mpu6050 (Autodesk Fusion 360 design; units mm, degrees)
Autodesk Fusion 360 part; units mm, degrees
sketch "Sketch1" plane through (0, 0, 0) normal (0, 0, 1) x (1, 0, 0)
  line L0 (-8.25, -9.75) -> (8.25, -9.75)
  line L1 (8.25, -9.75) -> (8.25, 9.75)
  line L2 (8.25, 9.75) -> (-8.25, 9.75)
  line L3 (-8.25, 9.75) -> (-8.25, -9.75)
  line L4 (-8.25, -9.75) -> (8.25, 9.75) construction
  line L5 (8.25, -9.75) -> (-8.25, 9.75) construction
  line L6 (-6.25, 9.75) -> (-6.25, -9.75) construction
  line L7 (-3.25, 9.75) -> (-3.25, -9.75) construction
  line L8 (-3.25, 0) -> (-6.25, 0) construction
  line L9 (-4.75, 7.25) -> (-4.75, -7.25) construction
  circle A0 centre (-4.75, 7.25) radius 1.5
  line L10 (-4.75, 7.25) -> (-4.75, 9.75) construction
  circle A1 centre (-4.75, -7.25) radius 1.5
  dimension "d1" = 16.5
  dimension "d2" = 19.5
  dimension "d3" = 2
  dimension "d4" = 3
  dimension "d5" = 2.5
  constraint horizontal L0
  constraint perpendicular L0 L1
  constraint parallel L0 L2
  constraint parallel L1 L3
  constraint coincident L4 origin
  constraint coincident L5 origin
  constraint coincident L2 L6.start
  constraint coincident L0 L6.end
  constraint perpendicular L0 L6
  constraint coincident L2 L7.start
  constraint coincident L0 L7.end
  constraint perpendicular L0 L7
  constraint midpoint L7 L8.start
  constraint midpoint L6 L8.end
  constraint perpendicular L8 L9
  constraint midpoint L8 L9
  constraint coincident L9.start A0.centre
  constraint tangent L6 A0
  constraint coincident L2 L10.end
  constraint perpendicular L2 L10
  constraint symmetric L8 A0 A1
  measures "d1" distance of L1.end L2.end
  measures "d2" distance of L0.end L1.end
  measures "d3" distance of L3 L6
  measures "d4" distance of L6 L7
  measures "d5" distance of L9.start L10.end
extrude "Extrude1" add sketch "Sketch1" along normal blind 2
sketch "Sketch2" plane through (0, 0, 2) normal (0, 0, 1) x (-1, 0, 0)
  circle A0 centre (4.75, 7.25) radius 1.5
  circle A1 centre (4.75, -7.25) radius 1.5
  line L0 (8.25, -9.75) -> (8.25, 9.75)
  line L1 (8.25, 9.75) -> (-8.25, 9.75)
  line L2 (-8.25, 9.75) -> (-8.25, -9.75)
  line L3 (-8.25, -9.75) -> (8.25, -9.75)
  line L4 (8.25, -9.4846) -> (-7.3185, -9.4846)
  line L5 (-7.3185, -9.4846) -> (-7.3185, 9.5005)
  line L6 (-7.3185, 9.5005) -> (8.25, 9.5005)
  line L7 (8.25, 9.5005) -> (8.25, -9.4846)
  constraint horizontal L4
  constraint vertical L5
  constraint horizontal L6
  constraint vertical L7
  constraint coincident L0 L4.start
extrude "Extrude2" cut sketch "Sketch2" against normal blind 20 contours L0 L1 L2 L3 L4 L5 L6
ref_plane "WorkPlane1" through (-0.4657, -0.0079, 3) normal (0, 0, 1) x (1, 0, 0)
sketch "Sketch3" plane through (-0.4657, -0.0079, 3) normal (0, 0, 1) x (1, 0, 0)
  line L0 (-0.2518, 1.7979, -1) -> (3.6711, 1.7979, -1)
  line L1 (3.6711, 1.7979, -1) -> (3.6711, -2.3324, -1)
  line L2 (3.6711, -2.3324, -1) -> (-0.2518, -2.3324, -1)
  line L3 (-0.2518, -2.3324, -1) -> (-0.2518, 1.7979, -1)
  line L4 (0.1158, 7.0063, -1) -> (1.8129, 7.0063, -1)
  line L5 (1.8129, 7.0063, -1) -> (1.8129, 4.1386, -1)
  line L6 (1.8129, 4.1386, -1) -> (0.1158, 4.1386, -1)
  line L7 (0.1158, 4.1386, -1) -> (0.1158, 7.0063, -1)
extrude "Extrude3" add sketch "Sketch3" along normal blind 1 contours L0 L1 L2 L3 | L4 L5 L6 L7 in plane through (-0.4657, -0.0079, 2) normal (0, 0, 1)
sketch "Sketch4" plane through (0, 0, 2) normal (0, 0, 1) x (-1, 0, 0)
  line L0 (0.7175, 2.3403) -> (0.7175, -1.7899)
  line L1 (0.7175, -1.7899) -> (-3.2053, -1.7899)
  line L2 (-3.2053, -1.7899) -> (-3.2053, 2.3403)
  line L3 (-3.2053, 2.3403) -> (0.7175, 2.3403)
  line L4 (0.3499, -4.1306) -> (0.3499, -6.9984)
  line L5 (0.3499, -6.9984) -> (-1.3472, -6.9984)
  line L6 (-1.3472, -6.9984) -> (-1.3472, -4.1306)
  line L7 (-1.3472, -4.1306) -> (0.3499, -4.1306)
  line L8 (8.25, 9.5005) -> (-7.3185, 9.5005)
  line L9 (-7.3185, 9.5005) -> (-7.3185, -9.4846)
  line L10 (-7.3185, -9.4846) -> (8.25, -9.4846)
  line L11 (8.25, -9.4846) -> (8.25, 9.5005)
  circle A0 centre (4.75, -7.25) radius 1.5
  circle A1 centre (4.75, 7.25) radius 1.5
  line L12 (8.25, -3.7805) -> (3.5552, -3.7805)
  line L13 (3.5552, -3.7805) -> (3.5552, 3.2297)
  line L14 (3.5552, 3.2297) -> (8.25, 3.2297)
  line L15 (8.25, 3.2297) -> (8.25, -3.7805)
  constraint horizontal L12
  constraint vertical L13
  constraint horizontal L14
  constraint vertical L15
  constraint coincident L11 L12.start
extrude "Extrude4" add sketch "Sketch4" along normal blind 3.5 contours L11 L12 L13 L14 L15
sketch "Sketch5" plane through (0, 0, 2) normal (0, 0, 1) x (-1, 0, 0)
  circle A0 centre (4.75, 7.25) radius 1.5
  circle A1 centre (4.75, -7.25) radius 1.5
  line L0 (8.25, -3.7805) -> (3.5552, -3.7805)
  line L1 (3.5552, -3.7805) -> (3.5552, 3.2297)
  line L2 (3.5552, 3.2297) -> (8.25, 3.2297)
  line L3 (8.25, 3.2297) -> (8.25, 9.5005)
  line L4 (8.25, 9.5005) -> (-7.3185, 9.5005)
  line L5 (-7.3185, 9.5005) -> (-7.3185, -9.4846)
  line L6 (-7.3185, -9.4846) -> (8.25, -9.4846)
  line L7 (8.25, -9.4846) -> (8.25, -3.7805)
  line L8 (0.3499, -4.1306) -> (0.3499, -6.9984)
  line L9 (0.3499, -6.9984) -> (-1.3472, -6.9984)
  line L10 (-1.3472, -6.9984) -> (-1.3472, -4.1306)
  line L11 (-1.3472, -4.1306) -> (0.3499, -4.1306)
  line L12 (0.7175, 2.3403) -> (0.7175, -1.7899)
  line L13 (0.7175, -1.7899) -> (-3.2053, -1.7899)
  line L14 (-3.2053, -1.7899) -> (-3.2053, 2.3403)
  line L15 (-3.2053, 2.3403) -> (0.7175, 2.3403)
  line L16 (-1.2611, 6.8567) -> (-3.3302, 6.8567)
  line L17 (-3.3302, 6.8567) -> (-3.3302, 7.6894)
  line L18 (-3.3302, 7.6894) -> (-1.2611, 7.6894)
  line L19 (-1.2611, 7.6894) -> (-1.2611, 6.8567)
  constraint horizontal L16
  constraint vertical L17
  constraint horizontal L18
  constraint vertical L19
extrude "Extrude5" add sketch "Sketch5" along normal blind 0.1 contours L16 L17 L18 L19
sketch "Sketch6" plane through (-8.25, 0, 0) normal (-1, 0, 0) x (0, -1, 0)
  line L0 (9.5005, 0) -> (9.5005, 2)
  line L1 (9.5005, 2) -> (3.2297, 2)
  line L2 (3.2297, 2) -> (3.2297, 5.5)
  line L3 (3.2297, 5.5) -> (-3.7805, 5.5)
  line L4 (-3.7805, 5.5) -> (-3.7805, 2)
  line L5 (-3.7805, 2) -> (-9.4846, 2)
  line L6 (-9.4846, 2) -> (-9.4846, 0)
  line L7 (-9.4846, 0) -> (9.5005, 0)
  line L8 (-3.7805, 2) -> (3.2297, 2)
  line L9 (-3.7805, 2.2) -> (3.2297, 2.2)
  dimension "d17" = -0.2
  constraint coincident L4.end L5.start
  constraint coincident L1.end L2.start
extrude "Extrude6" cut sketch "Sketch6" against normal blind 0.1 contours L2 L4 L8 L9
equation "d5 = d4 / 2 + 1 mm"
